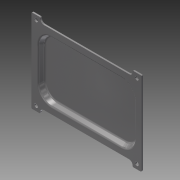
# Autodesk Inventor part: BoxLid
Saved by Autodesk Inventor 2014 SP2 (Build 180246200, 246)
## iProperties
Created: 2015-09-16
Part Number: BoxLid
Material: Steel, Galvanized
Document SubType Name: Modeling
Designer: Lukasz Szmit
Density: 7.85 g/cm^3
Appearance: Galvanized
Author: Lukasz Szmit
Autodesk Inventor part; units mm, degrees
ref_plane "YZ Plane" through (0, 0, 0) normal (1, 0, 0) x (0, 1, 0)
ref_plane "XZ Plane" through (0, 0, 0) normal (0, 1, 0) x (-1, 0, 0)
ref_plane "XY Plane" through (0, 0, 0) normal (0, 0, 1) x (1, 0, 0)
sketch "Sketch1" plane through (0, 0, 0) normal (0, 1, 0) x (-1, 0, 0)
  line L0 (-44.6422, 44.8224) -> (51.3578, 44.8224)
  line L1 (65.3578, 44.8224) -> (65.3578, -38.1776)
  line L2 (51.3578, -38.1776) -> (-44.6422, -38.1776)
  line L3 (-58.6422, -38.1776) -> (-58.6422, 44.8224)
  line L4 (65.3578, -38.1776) -> (65.3578, -42.6776)
  line L5 (64.3578, -43.6776) -> (56.3578, -43.6776)
  line L6 (55.3578, -42.6776) -> (55.3578, -42.1776)
  line L7 (-48.6422, -42.1776) -> (-48.6422, -42.6776)
  line L8 (-49.6422, -43.6776) -> (-57.6422, -43.6776)
  line L9 (-58.6422, -42.6776) -> (-58.6422, -38.1776)
  line L10 (55.3578, 48.8224) -> (55.3578, 49.3224)
  line L11 (56.3578, 50.3224) -> (64.3578, 50.3224)
  line L12 (65.3578, 49.3224) -> (65.3578, 44.8224)
  line L13 (-58.6422, 44.8224) -> (-58.6422, 49.3224)
  line L14 (-57.6422, 50.3224) -> (-49.6422, 50.3224)
  line L15 (-48.6422, 49.3224) -> (-48.6422, 48.8224)
  arc A0 (-48.6422, 48.8224) -> (-44.6422, 44.8224) centre (-44.6422, 48.8224) ccw
  arc A1 (51.3578, 44.8224) -> (55.3578, 48.8224) centre (51.3578, 48.8224) ccw
  arc A2 (-44.6422, -38.1776) -> (-48.6422, -42.1776) centre (-44.6422, -42.1776) ccw
  arc A3 (55.3578, -42.1776) -> (51.3578, -38.1776) centre (51.3578, -42.1776) ccw
  arc A4 (-58.6422, -42.6776) -> (-57.6422, -43.6776) centre (-57.6422, -42.6776) ccw
  arc A5 (-49.6422, -43.6776) -> (-48.6422, -42.6776) centre (-49.6422, -42.6776) ccw
  arc A6 (64.3578, -43.6776) -> (65.3578, -42.6776) centre (64.3578, -42.6776) ccw
  arc A7 (55.3578, -42.6776) -> (56.3578, -43.6776) centre (56.3578, -42.6776) ccw
  arc A8 (65.3578, 49.3224) -> (64.3578, 50.3224) centre (64.3578, 49.3224) ccw
  arc A9 (56.3578, 50.3224) -> (55.3578, 49.3224) centre (56.3578, 49.3224) ccw
  arc A10 (-57.6422, 50.3224) -> (-58.6422, 49.3224) centre (-57.6422, 49.3224) ccw
  arc A11 (-48.6422, 49.3224) -> (-49.6422, 50.3224) centre (-49.6422, 49.3224) ccw
  line L16 (51.3578, 44.8224) -> (41.1387, 44.8191)
  circle A12 centre (-53.4073, 45.0703) radius 2.25
  circle A13 centre (60.0919, 45.0669) radius 2.25
  arc A14 (65.3419, 49.3252) -> (64.3419, 50.3252) centre (64.3419, 49.3252) ccw
  circle A15 centre (-53.4081, -38.4248) radius 2.25
  circle A16 centre (60.0919, -38.428) radius 2.25
  line L17 (-58.6581, -31.6409) -> (-58.6581, -42.6748)
  point P0 (0, 0)
  point P1 (65.3578, -43.6776)
  point P2 (55.3578, -43.6776)
  point P3 (-48.6422, -43.6776)
  point P4 (-58.6422, -43.6776)
  point P5 (55.3578, 50.3224)
  point P6 (65.3578, 50.3224)
  point P7 (-58.6422, 50.3224)
  point P8 (-48.6422, 50.3224)
  point P9 (55.3578, 44.8224)
  point P10 (-48.6422, -38.1776)
  point P11 (49.6422, 43.6744)
  dimension "d0" = 83
  dimension "d1" = 5.5
  dimension "d2" = 5.5
  dimension "d3" = 10
  dimension "d4" = 5.5
  dimension "d5" = 10
  dimension "d6" = 5.5
  dimension "d7" = 94
  dimension "d8" = 1
  dimension "d9" = 124
  dimension "d10" = 96
  dimension "d11" = 90
  dimension "d15" = 5.25
  constraints: 36 end point, 26 point on circle, 24 tangent, 20 point on line, 17 centre point, 9 equal radius, 5 parallel, 2 perpendicular
  measures "d0" distance of L3.end L3.start
  measures "d1" distance of L1.end point (65.358, -43.678)
  measures "d2" distance of point (-48.642, -38.178) point (-48.642, -43.678)
  measures "d3" distance of point (55.358, 50.322) point (65.358, 50.322)
  measures "d4" distance of point (55.358, 44.822) point (55.358, 50.322)
  measures "d5" distance of point (-58.642, 50.322) point (-48.642, 50.322)
  measures "d6" distance of L3.end point (-58.642, 50.322)
  measures "d7" distance of point (-58.642, -43.678) point (-58.642, 50.322)
  measures "d8" radius of A4
  measures "d9" distance between parallel lines of L1 L3
  measures "d10" distance of L0.start L0.end
  measures "d11" angle of L2 L1
  measures "d15" distance from line of L17 A15.centre
extrude "Extrusion1" add sketch "Sketch1" along normal blind 2 contours L0 A1 L10 A9 L11 A8 L12 L1 L4 A6 L5 A7 L6 A3 L2 A2 L7 A5 L8 A4 L9 L3 L13 A10 L14 A11 L15 A0 | A12 | A13 | A15 | A16
ref_plane "Work Plane2" through (-56.3578, 2, -43.6776) normal (0, 1, 0) x (1, 0, 0)
sketch "Sketch4" plane through (-56.3578, 2, -43.6776) normal (0, 1, 0) x (1, 0, 0)
  circle A0 centre (-3.7506, -5.2942) radius 2.25
  circle A1 centre (109.7487, -5.2976) radius 2.25
  circle A2 centre (-3.7513, -88.7892) radius 2.25
  circle A3 centre (109.7487, -88.7925) radius 2.25
  constraints: 4 centre point
hole "Hole1" at (-60.1084, 2, -38.3834) at (-60.1091, 2, 45.1116) at (53.3909, 2, 45.1149) at (53.3909, 2, -38.38) direction (0, -1, 0) diameter 4 end through all
fillet "Fillet1" radius 0.5 24 edges at (-54.1862, 2, -39.3492) (-55.3578, 2, -42.4276) (-55.6507, 2, -43.3848) (-60.3578, 2, -43.6776) (-65.0649, 2, -43.3848) (-65.3578, 2, 3.3224) (-65.0649, 2, 50.0295) (-60.3578, 2, 50.3224) (-55.6507, 2, 50.0295) (-55.3578, 2, 49.0724) (-54.1862, 2, 45.9939) (-3.3578, 2, 44.8224) (47.4706, 2, 45.9939) (48.6422, 2, 49.0724) (48.9351, 2, 50.0295) (53.6422, 2, 50.3224) (58.3493, 2, 50.0295) (58.6422, 2, 3.3224) (58.3493, 2, -43.3848) (53.6422, 2, -43.6776) (48.9351, 2, -43.3848) (48.6422, 2, -42.4276) (47.4706, 2, -39.3492) (-3.3578, 2, -38.1776)
ref_plane "Work Plane3" through (0, 8, 0) normal (0, 1, 0) x (1, 0, 0)
sketch "Sketch6" plane through (0, 8, 0) normal (0, 1, 0) x (1, 0, 0)
  line L0 (-42.3578, 30.1776) -> (35.6422, 30.1776)
  line L1 (50.6422, 15.1776) -> (50.6422, -21.8224)
  line L2 (35.6422, -36.8224) -> (-42.3578, -36.8224)
  line L3 (-57.3578, -21.8224) -> (-57.3578, 15.1776)
  line L4 (44.6422, 38.1776) -> (-51.3578, 38.1776) projected
  line L5 (-65.3578, 42.6776) -> (-65.3578, -49.3224) projected
  line L6 (58.6422, -49.3224) -> (58.6422, 42.6776) projected
  line L7 (-51.3578, -44.8224) -> (44.6422, -44.8224) projected
  arc A0 (-42.3578, 30.1776) -> (-57.3578, 15.1776) centre (-42.3578, 15.1776) ccw
  arc A1 (50.6422, 15.1776) -> (35.6422, 30.1776) centre (35.6422, 15.1776) ccw
  arc A2 (35.6422, -36.8224) -> (50.6422, -21.8224) centre (35.6422, -21.8224) ccw
  arc A3 (-57.3578, -21.8224) -> (-42.3578, -36.8224) centre (-42.3578, -21.8224) ccw
  dimension "d69" = 8
  dimension "d70" = 8
  dimension "d71" = 8
  dimension "d72" = 8
  dimension "d73" = 15
  constraints: 8 end point, 8 point on circle, 8 tangent, 4 centre point, 3 equal radius
  measures "d69" distance between parallel lines of L4 L0
  measures "d70" distance between parallel lines of L5 L3
  measures "d71" distance between parallel lines of L6 L1
  measures "d72" distance between parallel lines of L7 L2
  measures "d73" radius of A0
sketch "Sketch7" plane through (-56.3578, 2, -43.6776) normal (0, 1, 0) x (1, 0, 0)
  line L0 (12, -11.5) -> (94, -11.5)
  line L1 (109, -26.5) -> (109, -67.5)
  line L2 (94, -82.5) -> (12, -82.5)
  line L3 (-3, -67.5) -> (-3, -26.5)
  arc A0 (12, -11.5) -> (-3, -26.5) centre (12, -26.5) ccw
  arc A1 (109, -26.5) -> (94, -11.5) centre (94, -26.5) ccw
  arc A2 (94, -82.5) -> (109, -67.5) centre (94, -67.5) ccw
  arc A3 (-3, -67.5) -> (12, -82.5) centre (12, -67.5) ccw
  line L4 (101, -5.5) -> (5, -5.5) projected
  line L5 (115, -93) -> (115, -1) projected
  line L6 (5, -88.5) -> (101, -88.5) projected
  line L7 (-9, -1) -> (-9, -93) projected
  dimension "d78" = 15
  dimension "d79" = 6
  dimension "d80" = 6
  dimension "d81" = 6
  dimension "d82" = 6
  constraints: 8 end point, 8 point on circle, 8 tangent, 4 centre point, 3 equal radius
  measures "d78" radius of A0
  measures "d79" distance between parallel lines of L4 L0
  measures "d80" distance between parallel lines of L5 L1
  measures "d81" distance between parallel lines of L6 L2
  measures "d82" distance between parallel lines of L7 L3
loft "Loft1" add profiles "Sketch7", "Sketch6"
ref_plane "Work Plane4" through (0, 6, 0) normal (0, 1, 0) x (1, 0, 0)
sketch "Sketch8" plane through (0, 6, 0) normal (0, 1, 0) x (1, 0, 0)
  line L0 (-40.8578, 28.6776) -> (34.1422, 28.6776)
  line L1 (49.1422, 13.6776) -> (49.1422, -20.3224)
  line L2 (34.1422, -35.3224) -> (-40.8578, -35.3224)
  line L3 (-55.8578, -20.3224) -> (-55.8578, 13.6776)
  arc A0 (-40.8578, 28.6776) -> (-55.8578, 13.6776) centre (-40.8578, 13.6776) ccw
  arc A1 (49.1422, 13.6776) -> (34.1422, 28.6776) centre (34.1422, 13.6776) ccw
  arc A2 (34.1422, -35.3224) -> (49.1422, -20.3224) centre (34.1422, -20.3224) ccw
  arc A3 (-55.8578, -20.3224) -> (-40.8578, -35.3224) centre (-40.8578, -20.3224) ccw
  line L4 (58.6422, -49.3224) -> (58.6422, 42.6776) projected
  line L5 (44.6422, 38.1776) -> (-51.3578, 38.1776) projected
  line L6 (-65.3578, 42.6776) -> (-65.3578, -49.3224) projected
  line L7 (-51.3578, -44.8224) -> (44.6422, -44.8224) projected
  dimension "d92" = 15
  dimension "d108" = 9.5
  dimension "d109" = 9.5
  dimension "d110" = 9.5
  dimension "d111" = 9.5
  constraints: 8 end point, 8 point on circle, 8 tangent, 4 centre point, 3 equal radius
  measures "d92" radius of A0
  measures "d108" distance between parallel lines of L4 L1
  measures "d109" distance between parallel lines of L5 L0
  measures "d110" distance between parallel lines of L6 L3
  measures "d111" distance between parallel lines of L7 L2
ref_plane "Work Plane5" through (-56.3578, 0, -43.6776) normal (0, 1, 0) x (1, 0, 0)
sketch "Sketch10" plane through (-56.3578, 0, -43.6776) normal (0, 1, 0) x (1, 0, 0)
  line L0 (13.5, -13) -> (92.5, -13)
  line L1 (107.5, -28) -> (107.5, -65.5)
  line L2 (92.5, -80.5) -> (13.5, -80.5)
  line L3 (-1.5, -65.5) -> (-1.5, -28)
  arc A0 (13.5, -13) -> (-1.5, -28) centre (13.5, -28) ccw
  arc A1 (107.5, -28) -> (92.5, -13) centre (92.5, -28) ccw
  arc A2 (92.5, -80.5) -> (107.5, -65.5) centre (92.5, -65.5) ccw
  arc A3 (-1.5, -65.5) -> (13.5, -80.5) centre (13.5, -65.5) ccw
  line L4 (101, -5.5) -> (5, -5.5) projected
  line L5 (-9, -1) -> (-9, -93) projected
  line L6 (115, -93) -> (115, -1) projected
  line L7 (101, -88) -> (5, -88) projected
  dimension "d99" = 15
  dimension "d112" = 7.5
  dimension "d113" = 7.5
  dimension "d114" = 7.5
  dimension "d115" = 7.5
  constraints: 8 end point, 8 point on circle, 8 tangent, 4 centre point, 3 equal radius
  measures "d99" radius of A0
  measures "d112" distance between parallel lines of L4 L0
  measures "d113" distance between parallel lines of L5 L3
  measures "d114" distance between parallel lines of L6 L1
  measures "d115" distance between parallel lines of L7 L2
loft "Loft2" cut profiles "Sketch10", "Sketch8"
fillet "Fillet2" radius 2 16 edges at (-52.9644, 8, -25.7842) (-57.3578, 8, 3.3224) (-52.9644, 8, 32.429) (-3.3578, 8, 36.8224) (46.2488, 8, 32.429) (50.6422, 8, 3.3224) (46.2488, 8, -25.7842) (-3.3578, 8, -30.1776) (-54.9644, 2, -27.7842) (-59.3578, 2, 3.3224) (-54.9644, 2, 34.429) (-3.3578, 2, 38.8224) (48.2488, 2, 34.429) (52.6422, 2, 3.3224) (48.2488, 2, -27.7842) (-3.3578, 2, -32.1776)
fillet "Fillet3" radius 2 16 edges at (-53.4644, 0, -26.2842) (-57.8578, 0, 3.0724) (-53.4644, 0, 32.429) (-3.3578, 0, 36.8224) (46.7488, 0, 32.429) (51.1422, 0, 3.0724) (46.7488, 0, -26.2842) (-3.3578, 0, -30.6776) (-51.4644, 6, -24.2842) (-55.8578, 6, 3.3224) (-51.4644, 6, 30.929) (-3.3578, 6, 35.3224) (44.7488, 6, 30.929) (49.1422, 6, 3.3224) (44.7488, 6, -24.2842) (-3.3578, 6, -28.6776)
body "Solid1"
